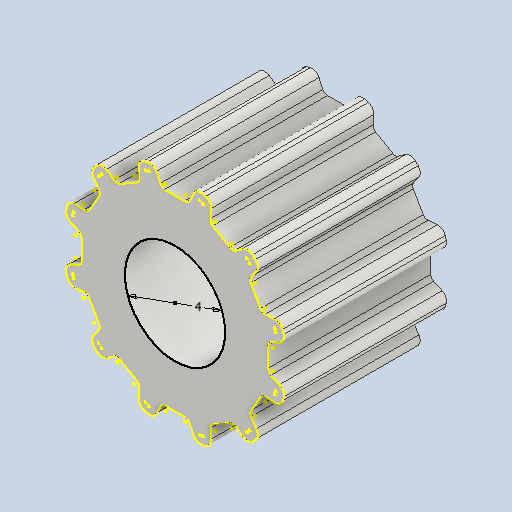
# Autodesk Inventor part: Synchronous Pulley1
Saved by Autodesk Inventor 2022.2 (Build 262287000, 287)
## iProperties
CustomPartVersion: 1
Created: 2022-01-04
Part Number: Synchronous Pulley1
Material: Steel
Document SubType Name: Modeling
Designer: Jochen
Density: 1 g/cm^3
Appearance: Steel
Author: Jochen
Autodesk Inventor part; units mm, degrees
ref_plane "YZ Plane" through (0, 0, 0) normal (1, 0, 0) x (0, 1, 0)
ref_plane "XZ Plane" through (0, 0, 0) normal (0, 1, 0) x (-1, 0, 0)
ref_plane "XY Plane" through (0, 0, 0) normal (0, 0, 1) x (1, 0, 0)
sketch "Pulley Sketch" plane through (0, 0, 0) normal (0, 0, 1) x (1, 0, 0)
  circle A0 centre (0, 0) radius 4.7746 construction
  circle A1 centre (0, 0) radius 4.4746
  circle A2 centre (0, 0) radius 3.7246
  line L0 (-0.8378, 4.3955) -> (-0.525, 3.7246)
  line L1 (-0.525, 3.7246) -> (0.525, 3.7246)
  line L2 (0.525, 3.7246) -> (0.8378, 4.3955)
  line L3 (0, 0) -> (0, 4.4746) construction
  point P0 (0, 3.7246)
  dimension "d0" = 9.5493
  dimension "d1" = 0.3
  dimension "d2" = 0.75
  dimension "d3" = 50
  dimension "d4" = 1.05
  constraints: 8 end point, 3 coincident, 3 point on circle, 2 centre point, 1 horizontal, 1 midpoint, 1 point on line, 1 vertical, 1 vertical alignment, 3 other
  measures "d0" diameter of A0
  measures "d1" radial gap between concentric circles of A0 A1
  measures "d3" angle of L2 L0
  measures "d4" distance of L0.end L1.end
extrude "Base Body" add sketch "Pulley Sketch" along normal mid plane 6 contours A2 | A1 L0 L1 L2 | L2 L1 L0 A1
extrude "Tooth" cut sketch "Pulley Sketch" along normal through all both and the other way through all contours L2 L1 L0 A1 picked at (0, 4.2187)
fillet "Tooth Fillet" radius 0.2 2 edges at (0.525, 3.7246, 0) (-0.525, 3.7246, 0)
fillet "Tooth Fillet" radius 0.3 4 edges at (-0.8378, 4.3955, 1.5) (-0.8378, 4.3955, -1.5) (0.8378, 4.3955, 1.5) (0.8378, 4.3955, -1.5)
pattern_circular "Teeth" count 12 over 360 about axis through (0, 0, -10) along (0, 0, 1) of "Tooth", "Tooth Fillet"
feature "Left flange" [suppressed]
feature "Right flange" [suppressed]
sketch "Sketch2" plane through (0, 0, 3) normal (0, 0, 1) x (1, 0, 0)
  arc A0 (0.3976, 3.7246) -> (0.5788, 3.8401) centre (0.3976, 3.9246) ccw projected
  line L0 (0.5788, 3.8401) -> (0.7363, 4.1779) projected
  arc A1 (1.0807, 4.3422) -> (0.7363, 4.1779) centre (1.0082, 4.0511) ccw projected
  arc A2 (1.2352, 4.3008) -> (1.0807, 4.3422) centre (0, 0) ccw projected
  arc A3 (1.4512, 3.9863) -> (1.2352, 4.3008) centre (1.1524, 4.0124) ccw projected
  line L1 (1.4512, 3.9863) -> (1.4188, 3.6151) projected
  arc A4 (1.4188, 3.6151) -> (1.518, 3.4244) centre (1.618, 3.5976) ccw projected
  line L2 (1.518, 3.4244) -> (2.2066, 3.0268) projected
  arc A5 (2.2066, 3.0268) -> (2.4214, 3.0362) centre (2.3066, 3.2001) ccw projected
  line L3 (2.4214, 3.0362) -> (2.7266, 3.25) projected
  arc A6 (3.107, 3.2201) -> (2.7266, 3.25) centre (2.8987, 3.0042) ccw projected
  arc A7 (3.2201, 3.107) -> (3.107, 3.2201) centre (0, 0) ccw projected
  arc A8 (3.25, 2.7266) -> (3.2201, 3.107) centre (3.0042, 2.8987) ccw projected
  line L4 (3.25, 2.7266) -> (3.0362, 2.4214) projected
  arc A9 (3.0362, 2.4214) -> (3.0268, 2.2066) centre (3.2001, 2.3066) ccw projected
  line L5 (3.0268, 2.2066) -> (3.4244, 1.518) projected
  arc A10 (3.4244, 1.518) -> (3.6151, 1.4188) centre (3.5976, 1.618) ccw projected
  line L6 (3.6151, 1.4188) -> (3.9863, 1.4512) projected
  arc A11 (4.3008, 1.2352) -> (3.9863, 1.4512) centre (4.0124, 1.1524) ccw projected
  arc A12 (4.3422, 1.0807) -> (4.3008, 1.2352) centre (0, 0) ccw projected
  arc A13 (4.1779, 0.7363) -> (4.3422, 1.0807) centre (4.0511, 1.0082) ccw projected
  line L7 (4.1779, 0.7363) -> (3.8401, 0.5788) projected
  arc A14 (3.8401, 0.5788) -> (3.7246, 0.3976) centre (3.9246, 0.3976) ccw projected
  line L8 (3.7246, 0.3976) -> (3.7246, -0.3976) projected
  arc A15 (3.7246, -0.3976) -> (3.8401, -0.5788) centre (3.9246, -0.3976) ccw projected
  line L9 (3.8401, -0.5788) -> (4.1779, -0.7363) projected
  arc A16 (4.3422, -1.0807) -> (4.1779, -0.7363) centre (4.0511, -1.0082) ccw projected
  arc A17 (4.3008, -1.2352) -> (4.3422, -1.0807) centre (0, 0) ccw projected
  arc A18 (3.9863, -1.4512) -> (4.3008, -1.2352) centre (4.0124, -1.1524) ccw projected
  line L10 (3.9863, -1.4512) -> (3.6151, -1.4188) projected
  arc A19 (3.6151, -1.4188) -> (3.4244, -1.518) centre (3.5976, -1.618) ccw projected
  line L11 (3.4244, -1.518) -> (3.0268, -2.2066) projected
  arc A20 (3.0268, -2.2066) -> (3.0362, -2.4214) centre (3.2001, -2.3066) ccw projected
  line L12 (3.0362, -2.4214) -> (3.25, -2.7266) projected
  arc A21 (3.2201, -3.107) -> (3.25, -2.7266) centre (3.0042, -2.8987) ccw projected
  arc A22 (3.107, -3.2201) -> (3.2201, -3.107) centre (0, 0) ccw projected
  arc A23 (2.7266, -3.25) -> (3.107, -3.2201) centre (2.8987, -3.0042) ccw projected
  line L13 (2.7266, -3.25) -> (2.4214, -3.0362) projected
  arc A24 (2.4214, -3.0362) -> (2.2066, -3.0268) centre (2.3066, -3.2001) ccw projected
  line L14 (2.2066, -3.0268) -> (1.518, -3.4244) projected
  arc A25 (1.518, -3.4244) -> (1.4188, -3.6151) centre (1.618, -3.5976) ccw projected
  line L15 (1.4188, -3.6151) -> (1.4512, -3.9863) projected
  arc A26 (1.2352, -4.3008) -> (1.4512, -3.9863) centre (1.1524, -4.0124) ccw projected
  arc A27 (1.0807, -4.3422) -> (1.2352, -4.3008) centre (0, 0) ccw projected
  arc A28 (0.7363, -4.1779) -> (1.0807, -4.3422) centre (1.0082, -4.0511) ccw projected
  line L16 (0.7363, -4.1779) -> (0.5788, -3.8401) projected
  arc A29 (0.5788, -3.8401) -> (0.3976, -3.7246) centre (0.3976, -3.9246) ccw projected
  line L17 (0.3976, -3.7246) -> (-0.3976, -3.7246) projected
  arc A30 (-0.3976, -3.7246) -> (-0.5788, -3.8401) centre (-0.3976, -3.9246) ccw projected
  line L18 (-0.5788, -3.8401) -> (-0.7363, -4.1779) projected
  arc A31 (-1.0807, -4.3422) -> (-0.7363, -4.1779) centre (-1.0082, -4.0511) ccw projected
  arc A32 (-1.2352, -4.3008) -> (-1.0807, -4.3422) centre (0, 0) ccw projected
  arc A33 (-1.4512, -3.9863) -> (-1.2352, -4.3008) centre (-1.1524, -4.0124) ccw projected
  line L19 (-1.4512, -3.9863) -> (-1.4188, -3.6151) projected
  arc A34 (-1.4188, -3.6151) -> (-1.518, -3.4244) centre (-1.618, -3.5976) ccw projected
  line L20 (-1.518, -3.4244) -> (-2.2066, -3.0268) projected
  arc A35 (-2.2066, -3.0268) -> (-2.4214, -3.0362) centre (-2.3066, -3.2001) ccw projected
  line L21 (-2.4214, -3.0362) -> (-2.7266, -3.25) projected
  arc A36 (-3.107, -3.2201) -> (-2.7266, -3.25) centre (-2.8987, -3.0042) ccw projected
  arc A37 (-3.2201, -3.107) -> (-3.107, -3.2201) centre (0, 0) ccw projected
  arc A38 (-3.25, -2.7266) -> (-3.2201, -3.107) centre (-3.0042, -2.8987) ccw projected
  line L22 (-3.25, -2.7266) -> (-3.0362, -2.4214) projected
  arc A39 (-3.0362, -2.4214) -> (-3.0268, -2.2066) centre (-3.2001, -2.3066) ccw projected
  line L23 (-3.0268, -2.2066) -> (-3.4244, -1.518) projected
  arc A40 (-3.4244, -1.518) -> (-3.6151, -1.4188) centre (-3.5976, -1.618) ccw projected
  line L24 (-3.6151, -1.4188) -> (-3.9863, -1.4512) projected
  arc A41 (-4.3008, -1.2352) -> (-3.9863, -1.4512) centre (-4.0124, -1.1524) ccw projected
  arc A42 (-4.3422, -1.0807) -> (-4.3008, -1.2352) centre (0, 0) ccw projected
  arc A43 (-4.1779, -0.7363) -> (-4.3422, -1.0807) centre (-4.0511, -1.0082) ccw projected
  line L25 (-4.1779, -0.7363) -> (-3.8401, -0.5788) projected
  arc A44 (-3.8401, -0.5788) -> (-3.7246, -0.3976) centre (-3.9246, -0.3976) ccw projected
  line L26 (-3.7246, -0.3976) -> (-3.7246, 0.3976) projected
  arc A45 (-3.7246, 0.3976) -> (-3.8401, 0.5788) centre (-3.9246, 0.3976) ccw projected
  line L27 (-3.8401, 0.5788) -> (-4.1779, 0.7363) projected
  arc A46 (-4.3422, 1.0807) -> (-4.1779, 0.7363) centre (-4.0511, 1.0082) ccw projected
  arc A47 (-4.3008, 1.2352) -> (-4.3422, 1.0807) centre (0, 0) ccw projected
  arc A48 (-3.9863, 1.4512) -> (-4.3008, 1.2352) centre (-4.0124, 1.1524) ccw projected
  line L28 (-3.9863, 1.4512) -> (-3.6151, 1.4188) projected
  arc A49 (-3.6151, 1.4188) -> (-3.4244, 1.518) centre (-3.5976, 1.618) ccw projected
  line L29 (-3.4244, 1.518) -> (-3.0268, 2.2066) projected
  arc A50 (-3.0268, 2.2066) -> (-3.0362, 2.4214) centre (-3.2001, 2.3066) ccw projected
  line L30 (-3.0362, 2.4214) -> (-3.25, 2.7266) projected
  arc A51 (-3.2201, 3.107) -> (-3.25, 2.7266) centre (-3.0042, 2.8987) ccw projected
  arc A52 (-3.107, 3.2201) -> (-3.2201, 3.107) centre (0, 0) ccw projected
  arc A53 (-2.7266, 3.25) -> (-3.107, 3.2201) centre (-2.8987, 3.0042) ccw projected
  line L31 (-2.7266, 3.25) -> (-2.4214, 3.0362) projected
  arc A54 (-2.4214, 3.0362) -> (-2.2066, 3.0268) centre (-2.3066, 3.2001) ccw projected
  line L32 (-2.2066, 3.0268) -> (-1.518, 3.4244) projected
  arc A55 (-1.518, 3.4244) -> (-1.4188, 3.6151) centre (-1.618, 3.5976) ccw projected
  line L33 (-1.4188, 3.6151) -> (-1.4512, 3.9863) projected
  arc A56 (-1.2352, 4.3008) -> (-1.4512, 3.9863) centre (-1.1524, 4.0124) ccw projected
  arc A57 (-1.0807, 4.3422) -> (-1.2352, 4.3008) centre (0, 0) ccw projected
  arc A58 (-0.7363, 4.1779) -> (-1.0807, 4.3422) centre (-1.0082, 4.0511) ccw projected
  line L34 (-0.7363, 4.1779) -> (-0.5788, 3.8401) projected
  arc A59 (-0.5788, 3.8401) -> (-0.3976, 3.7246) centre (-0.3976, 3.9246) ccw projected
  line L35 (-0.3976, 3.7246) -> (0.3976, 3.7246) projected
  circle A60 centre (0, 0) radius 2
  dimension "d17" = 4
  constraints: 1 centre point, 1 coincident
  measures "d17" diameter of A60
extrude "Extrusion3" cut sketch "Sketch2" along normal through all both and the other way through all contours A60
extrude "Extrusion5" add sketch "Sketch2" against normal blind 0.5 from surface at -6
equation "\"d1\" = da_a"
equation "\"d2\" = da_hg"
equation "\"d3\" = 2 * da_fi"
equation "\"d4\" = da_bw"
equation "\"d5\" = da_bf"
equation "\"d7\" = da_bf"
equation "\"d9\" = da_rb"
equation "\"d10\" = da_rt"
equation "\"da_pb\" = 2.5"
equation "\"da_fi\" = 25deg"
equation "\"da_hg\" = 0.75"
equation "\"da_bw\" = 1.05"
equation "\"da_rb\" = 0.2"
equation "\"da_rt\" = 0.3"
equation "\"da_a\" = 0.3"
equation "\"da_bf\" = 6"
equation "\"da_wf\" = 1.5"
equation "\"da_hf\" = 1.5"
body "Solid1"
